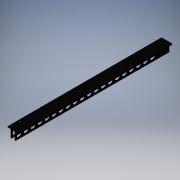
# Autodesk Inventor part: Arm_light
Saved by Autodesk Inventor 2016 (Build 200138000, 138)
## iProperties
Created: 2015-09-09
Part Number: Arm_light
Material: Aluminum 6061
Document SubType Name: Modeling
Designer: Dima
Density: 2.7 g/cm^3
Appearance: Anodized - Black
Author: Dima
Autodesk Inventor part; units mm, degrees
ref_plane "YZ Plane" through (0, 0, 0) normal (1, 0, 0) x (0, 1, 0)
ref_plane "XZ Plane" through (0, 0, 0) normal (0, 1, 0) x (-1, 0, 0)
ref_plane "XY Plane" through (0, 0, 0) normal (0, 0, 1) x (1, 0, 0)
sketch "Sketch1" plane through (0, 0, 0) normal (0, 0, 1) x (1, 0, 0)
  line L0 (0, 0) -> (17.526, 0)
  line L1 (17.526, 0) -> (17.526, -1.524)
  line L2 (17.526, -1.524) -> (12.7762, -1.524)
  line L3 (12.7762, -1.524) -> (12.7762, -14.351)
  line L4 (12.7762, -14.351) -> (11.2522, -14.351)
  line L5 (11.2522, -14.351) -> (11.2522, -1.524)
  line L6 (11.2522, -1.524) -> (6.2738, -1.524)
  line L7 (6.2738, -1.524) -> (6.2738, -14.351)
  line L8 (6.2738, -14.351) -> (4.7498, -14.351)
  line L9 (4.7498, -14.351) -> (4.7498, -1.524)
  line L10 (4.7498, -1.524) -> (0, -1.524)
  line L11 (0, -1.524) -> (0, 0)
  dimension "d0" = 17.526
  dimension "d1" = 1.524
  dimension "d2" = 4.7498
  dimension "d3" = 12.827
  dimension "d4" = 1.524
  dimension "d5" = 4.9784
  dimension "d6" = 1.524
  constraints: 24 end point, 5 parallel, 5 perpendicular, 1 collinear, 1 horizontal
  measures "d0" distance of L0.start L0.end
  measures "d1" distance of L0.end L1.end
  measures "d2" distance of L1.end L2.end
  measures "d3" distance of L2.end L3.end
  measures "d4" distance of L3.end L4.end
  measures "d5" distance of L5.end L6.end
  measures "d6" distance of L7.end L8.end
extrude "Extrusion1" add sketch "Sketch1" against normal blind 249.9995
sketch "Sketch2" plane through (0, 0, 0) normal (0, 1, 0) x (1, 0, 0)
  line L0 (0, 0) -> (17.526, 0) projected
  line L1 (0, 0) -> (0, 249.9995) projected
  line L2 (8.763, 0) -> (8.763, 10.16)
  circle A0 centre (8.763, 10.16) radius 2.413
  circle A1 centre (8.763, 10.16) radius 9.5
  circle A2 centre (8.763, 10.16) radius 8
  line L3 (8.763, 10.16) -> (2.6565, 17.4374)
  line L4 (8.763, 10.16) -> (18.263, 10.16) construction
  line L5 (8.763, 10.16) -> (14.8695, 2.8826)
  line L6 (8.763, 10.16) -> (2.6346, 5.0177)
  line L7 (8.763, 10.16) -> (14.8914, 15.3023)
  circle A3 centre (2.6346, 5.0177) radius 1.5
  circle A4 centre (2.6565, 17.4374) radius 1.5
  circle A5 centre (14.8914, 15.3023) radius 1.5
  circle A6 centre (14.8695, 2.8826) radius 1.5
  dimension "d9" = 10.16
  dimension "d10" = 4.826
  dimension "d11" = 19
  dimension "d12" = 16
  dimension "d13" = 130
  dimension "d14" = 3
  dimension "d15" = 3
  dimension "d16" = 3
  dimension "d17" = 3
  constraints: 12 end point, 7 centre point, 7 coincident, 4 point on circle, 2 collinear, 1 equal length, 1 horizontal, 1 midpoint, 1 parallel, 1 perpendicular
  measures "d9" distance of L2.start L2.end
  measures "d10" diameter of A0
  measures "d11" diameter of A1
  measures "d12" diameter of A2
  measures "d13" angle of L4 L3
  measures "d14" diameter of A3
  measures "d15" diameter of A4
  measures "d16" diameter of A5
  measures "d17" diameter of A6
extrude "Extrusion2" cut sketch "Sketch2" against normal blind 1.524 contours A3 A2 | A6 L5 A1 | A1 A6 | A4 A1 | A1 L3 A4 | A3 L6 A2 | A2 L6 A3 | A0 L6 L2 | L2 L5 A0 | A6 A1 L5 | A1 A4 L3 | L6 A0 L3 | L7 A0 L5 | L3 A0 L7 | A5 A2 | A2 L7 A5 | A5 L7 A2
sketch "Sketch3" plane through (0, 0, 0) normal (0, 1, 0) x (1, 0, 0)
  line L0 (0, 249.9995) -> (17.526, 249.9995) projected
  line L1 (0, 0) -> (0, 249.9995) projected
  line L2 (8.763, 249.9995) -> (8.763, 244.6655)
  line L3 (8.763, 244.6655) -> (8.763, 234.6579)
  circle A0 centre (8.763, 244.6655) radius 1.5
  circle A1 centre (8.763, 234.6579) radius 1.5
  dimension "d20" = 5.334
  dimension "d21" = 10.0076
  dimension "d22" = 3
  dimension "d23" = 3
  constraints: 4 end point, 2 centre point, 2 coincident, 1 collinear, 1 midpoint, 1 parallel
  measures "d20" distance of L2.start L2.end
  measures "d21" distance of L2.end L3.end
  measures "d22" diameter of A0
  measures "d23" diameter of A1
extrude "Extrusion3" cut sketch "Sketch3" against normal blind 1.524
sketch "Sketch5" plane through (12.7762, -14.351, 0) normal (1, 0, 0) x (0, 0, -1)
  line L0 (0, 12.827) -> (0, 0) projected
  line L1 (0, 0) -> (249.9995, 0) projected
  line L2 (0, 12.827) -> (249.9995, 12.827) projected
  line L3 (0, 6.4135) -> (6.4262, 6.4135)
  circle A0 centre (6.4262, 6.4135) radius 4.445
  circle A1 centre (17.8562, 6.4135) radius 4.445
  circle A2 centre (29.2862, 6.4135) radius 4.445
  circle A3 centre (40.7162, 6.4135) radius 4.445
  circle A4 centre (52.1462, 6.4135) radius 4.445
  circle A5 centre (63.5762, 6.4135) radius 4.445
  circle A6 centre (75.0062, 6.4135) radius 4.445
  circle A7 centre (86.4362, 6.4135) radius 4.445
  circle A8 centre (97.8662, 6.4135) radius 4.445
  circle A9 centre (109.2962, 6.4135) radius 4.445
  circle A10 centre (120.7262, 6.4135) radius 4.445
  circle A11 centre (132.1562, 6.4135) radius 4.445
  circle A12 centre (143.5862, 6.4135) radius 4.445
  circle A13 centre (155.0162, 6.4135) radius 4.445
  circle A14 centre (166.4462, 6.4135) radius 4.445
  circle A15 centre (177.8762, 6.4135) radius 4.445
  circle A16 centre (189.3062, 6.4135) radius 4.445
  circle A17 centre (200.7362, 6.4135) radius 4.445
  circle A18 centre (212.1662, 6.4135) radius 4.445
  circle A19 centre (223.5962, 6.4135) radius 4.445
  point P0 (0, 14.351)
  dimension "d38" = 6.4262
  dimension "d39" = 8.89
  dimension "d42" = 11.43
  constraints: 20 centre point, 2 end point, 1 coincident, 1 horizontal, 1 midpoint, 1 parallel, 38 other
  measures "d38" distance of L3.start L3.end
  measures "d39" diameter of A0
  measures "d42" distance of A0.centre A1.centre
extrude "Extrusion4" cut sketch "Sketch5" against normal blind 25.4
body "Solid1"
